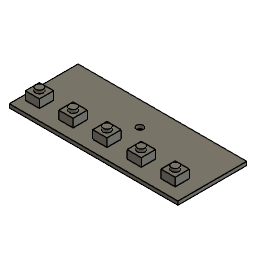
Плата кнопок (Autodesk Fusion 360 design; units mm, degrees)
part number: 2026-08-15-16-35-27-708
Autodesk Fusion 360 part; units mm, degrees
sketch "Эскиз1" plane through (0, 0, 0) normal (0, 1, 0) x (1, 0, 0)
  line L0 (36.85, -15.05) -> (-36.85, -15.05)
  line L1 (-36.85, -15.05) -> (-36.85, 15.05)
  line L2 (-36.85, 15.05) -> (36.85, 15.05)
  line L3 (36.85, 15.05) -> (36.85, -15.05)
  line L4 (36.85, -15.05) -> (-36.85, 15.05) construction
  line L5 (-36.85, -15.05) -> (36.85, 15.05) construction
  circle A0 centre (0.65, 4.55) radius 1.5
  dimension "d1" = 73.7
  dimension "d2" = 30.1
  dimension "d3" = 3
  dimension "d4" = 37.5
  dimension "d5" = 10.5
  constraint horizontal L0
  constraint perpendicular L0 L1
  constraint parallel L0 L2
  constraint parallel L1 L3
  constraint coincident L4 origin
  constraint coincident L5 origin
  measures "d1" distance of L1.end L2.end
  measures "d2" distance of L0.end L1.end
  measures "d3" diameter of A0
  measures "d4" distance of L1 A0.centre
  measures "d5" distance of L2 A0.centre
extrude "Выдавливание2" add sketch "Эскиз1" along normal blind 1.6
sketch "Эскиз2" plane through (0, 1.6, 0) normal (0, 1, 0) x (-1, 0, 0)
  line L0 (34.65, 4.05) -> (28.45, 4.05)
  line L1 (28.45, 4.05) -> (28.45, 10.25)
  line L2 (28.45, 10.25) -> (34.65, 10.25)
  line L3 (34.65, 10.25) -> (34.65, 4.05)
  circle A0 centre (-0.65, -4.55) radius 1.5
  circle A1 centre (-0.65, -4.55) radius 1.5
  line L4 (-36.85, -15.05) -> (36.85, -15.05)
  line L5 (36.85, -15.05) -> (36.85, 15.05)
  line L6 (36.85, 15.05) -> (-36.85, 15.05)
  line L7 (-36.85, 15.05) -> (-36.85, -15.05)
  line L8 (19.95, 4.05) -> (13.75, 4.05)
  line L9 (19.95, 10.25) -> (19.95, 4.05)
  line L10 (13.75, 10.25) -> (19.95, 10.25)
  line L11 (13.75, 4.05) -> (13.75, 10.25)
  line L12 (5.15, 4.05) -> (-1.05, 4.05)
  line L13 (5.15, 10.25) -> (5.15, 4.05)
  line L14 (-1.05, 10.25) -> (5.15, 10.25)
  line L15 (-1.05, 4.05) -> (-1.05, 10.25)
  line L16 (-9.85, 4.05) -> (-16.05, 4.05)
  line L17 (-9.85, 10.25) -> (-9.85, 4.05)
  line L18 (-16.05, 4.05) -> (-16.05, 10.25)
  line L19 (-16.05, 10.25) -> (-9.85, 10.25)
  line L20 (-24.65, 4.05) -> (-30.85, 4.05)
  line L21 (-24.65, 10.25) -> (-24.65, 4.05)
  line L22 (-30.85, 4.05) -> (-30.85, 10.25)
  line L23 (-30.85, 10.25) -> (-24.65, 10.25)
  dimension "d8" = 6.2
  dimension "d9" = 6.2
  dimension "d18" = 2.2
  dimension "d19" = 4.8
  dimension "d20" = 6.2
  dimension "d21" = 6.2
  dimension "d22" = 8.5
  dimension "d23" = 6.2
  dimension "d24" = 6.2
  dimension "d25" = 8.6
  dimension "d26" = 6.2
  dimension "d27" = 6.2
  dimension "d28" = 6.2
  dimension "d29" = 6.2
  dimension "d30" = 8.6
  dimension "d31" = 8.8
  dimension "d32" = 65.5
  dimension "d33" = 21
  dimension "d34" = 21.2
  dimension "d35" = 21
  dimension "d36" = 20.9
  dimension "d37" = 6
  constraint horizontal L0
  constraint vertical L1
  constraint horizontal L2
  constraint vertical L3
  constraint horizontal L8
  constraint vertical L11
  constraint horizontal L10
  constraint vertical L9
  constraint horizontal L12
  constraint vertical L15
  constraint horizontal L14
  constraint vertical L13
  constraint horizontal L16
  constraint vertical L18
  constraint horizontal L19
  constraint vertical L17
  constraint horizontal L20
  constraint vertical L22
  constraint horizontal L23
  constraint vertical L21
  measures "d8" distance of L0.start L0.end
  measures "d9" distance of L0.start L2.end
  measures "d18" distance of L3 L5
  measures "d19" distance of L2 L6
  measures "d20" distance of L8.start L8.end
  measures "d21" distance of L9.start L8.start
  measures "d22" distance of L1 L9
  measures "d23" distance of L12.start L12.end
  measures "d24" distance of L13.start L12.start
  measures "d25" distance of L11 L13
  measures "d26" distance of L16.start L16.end
  measures "d27" distance of L17.start L16.start
  measures "d28" distance of L20.end L20.start
  measures "d29" distance of L21.start L20.start
  measures "d30" distance of L18 L21
  measures "d31" distance of L15 L17
  measures "d32" distance of L3 L22
  measures "d33" distance of L17 L22
  measures "d34" distance of L13 L18
  measures "d35" distance of L9 L15
  measures "d36" distance of L3 L11
  measures "d37" distance of L7 L22
extrude "Выдавливание3" add sketch "Эскиз2" along normal blind 3.6 contours L0 L1 L2 L3 | L8 L9 L10 L11 | L12 L13 L14 L15 | L16 L17 L18 L19 | L20 L21 L22 L23
sketch "Эскиз3" plane through (0, 5.2, 0) normal (0, 1, 0) x (-1, 0, 0)
  line L0 (34.65, 10.25) -> (28.45, 10.25)
  line L1 (28.45, 10.25) -> (28.45, 4.05)
  line L2 (28.45, 4.05) -> (34.65, 4.05)
  line L3 (34.65, 4.05) -> (34.65, 10.25)
  line L4 (13.75, 4.05) -> (19.95, 4.05)
  line L5 (19.95, 4.05) -> (19.95, 10.25)
  line L6 (19.95, 10.25) -> (13.75, 10.25)
  line L7 (13.75, 10.25) -> (13.75, 4.05)
  line L8 (-1.05, 4.05) -> (5.15, 4.05)
  line L9 (5.15, 4.05) -> (5.15, 10.25)
  line L10 (5.15, 10.25) -> (-1.05, 10.25)
  line L11 (-1.05, 10.25) -> (-1.05, 4.05)
  line L12 (-16.05, 10.25) -> (-16.05, 4.05)
  line L13 (-16.05, 4.05) -> (-9.85, 4.05)
  line L14 (-9.85, 4.05) -> (-9.85, 10.25)
  line L15 (-9.85, 10.25) -> (-16.05, 10.25)
  line L16 (-30.85, 10.25) -> (-30.85, 4.05)
  line L17 (-30.85, 4.05) -> (-24.65, 4.05)
  line L18 (-24.65, 4.05) -> (-24.65, 10.25)
  line L19 (-24.65, 10.25) -> (-30.85, 10.25)
  circle A0 centre (31.55, 7.15) radius 1.7
  circle A1 centre (16.85, 7.15) radius 1.7
  circle A2 centre (2.05, 7.15) radius 1.7
  circle A3 centre (-12.95, 7.15) radius 1.7
  circle A4 centre (-27.75, 7.15) radius 1.7
  dimension "d40" = 3.4
  dimension "d41" = 3.4
  dimension "d42" = 3.4
  dimension "d43" = 3.4
  dimension "d44" = 3.4
  measures "d40" diameter of A0
  measures "d41" diameter of A1
  measures "d42" diameter of A2
  measures "d43" diameter of A3
  measures "d44" diameter of A4
extrude "Выдавливание4" add sketch "Эскиз3" along normal blind 1.4 contours A0 | A1 | A2 | A3 | A4
